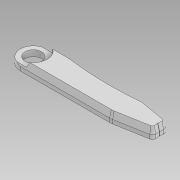
# Autodesk Inventor part: DoubleSlipHR_Bar
Saved by Autodesk Inventor 2021 (Build 250183000, 183)
## iProperties
Created: 2021-05-06
Part Number: DoubleSlipHR_Bar
Material: 一般
Document SubType Name: Modeling
Designer: kumagai
Density: 1 g/cm^3
Appearance: 既定
Author: kumagai
Autodesk Inventor part; units mm, degrees
ref_plane "YZ Plane" through (0, 0, 0) normal (1, 0, 0) x (0, 1, 0)
ref_plane "XZ Plane" through (0, 0, 0) normal (0, 1, 0) x (-1, 0, 0)
ref_plane "XY Plane" through (0, 0, 0) normal (0, 0, 1) x (1, 0, 0)
derived "DoubleSlipHR.ipt"
sketch "スケッチ1" plane through (0, 0, 0) normal (0, 1, 0) x (-1, 0, 0)
  line L0 (0, -123.3522) -> (0, 25.2475) projected
  line L1 (-47.4955, 0) -> (12.5826, 0) projected
  circle A0 centre (0, 0) radius 2.525
  circle A1 centre (0, 0) radius 4
  line L2 (0, 4) -> (-27.2419, 4)
  line L3 (-38.5128, 1.1628) -> (-38.4149, 0.0436)
  line L4 (-38.4149, -0.0436) -> (-38.5128, -1.1628)
  arc A2 (-38.4149, -0.0436) -> (-38.4149, 0.0436) centre (-38.913, 0) ccw
  arc A3 (-7.5002, -3.9826) -> (-29.3884, -3.5223) centre (-20.513, -102.1237) ccw
  line L5 (-31.474, 0) -> (-33.3295, 0)
  line L6 (0, -4) -> (-7.2374, -4)
  line L7 (-30.7049, -3.4665) -> (-37.6902, -2.2348)
  line L8 (-28.1101, 3.924) -> (-37.6902, 2.2348)
  arc A4 (-38.5128, -1.1628) -> (-37.6902, -2.2348) centre (-37.5166, -1.25) ccw
  arc A5 (-37.6902, 2.2348) -> (-38.5128, 1.1628) centre (-37.5166, 1.25) ccw
  arc A6 (-27.2419, 4) -> (-28.1101, 3.924) centre (-27.2419, -1) ccw
  arc A7 (-30.7049, -3.4665) -> (-29.3884, -3.5223) centre (-29.8366, 1.4575) ccw
  arc A8 (-7.5002, -3.9826) -> (-7.2374, -4) centre (-7.2374, -2) ccw
  point P0 (-38.411, 0)
  point P1 (-38.5278, -1.3348)
  point P2 (-38.4707, -0.6822)
  point P3 (-38.413, 0)
  point P4 (-31.0718, 4)
  point P5 (-7.37, -4)
  dimension "d1" = 5.05
  dimension "d2" = 8
  dimension "d4" = 0.5
  dimension "d7" = 170
  dimension "d9" = 38.413
  dimension "d14" = 20.513
  dimension "d15" = 102.1237
  dimension "d17" = 0
  dimension "d18" = 99
  dimension "d27" = 20
  dimension "d28" = 1
  dimension "d29" = 2.5
  dimension "d30" = 5
  dimension "d31" = 5
  dimension "d39" = 2
  constraints: 18 point on circle, 14 end point, 12 tangent, 10 point on line, 9 centre point, 3 horizontal, 2 coincident, 1 equal radius, 2 other
  measures "d1" diameter of A0
  measures "d2" diameter of A1
  measures "d4" radius of A2
  measures "d7" angle of L3 L4
  measures "d9" distance from line of point (-38.413, 0) L0
  measures "d14" distance from line of L0 A3.centre
  measures "d15" distance from line of L1 A3.centre
  measures "d17" distance between parallel lines of L1 L5
  measures "d18" radius of A3
  measures "d27" angle of L8 L7
  measures "d28" radius of A4
  measures "d29" distance of A5.centre A4.centre
  measures "d30" radius of A6
  measures "d31" radius of A7
  measures "d39" radius of A8
extrude "押し出し1" add sketch "スケッチ1" along normal blind 3.2 contours A1 L1 A0 L0 | L0 A0 L1 A1 | L6 A8 A3 A7 L7 A4 L4 A2 L1 A1 | L1 A0 L0 A1 | A1 L0 A0 L1 | L1 A2 L3 A5 L8 A6 L2 A1
sketch "スケッチ2" plane through (0, 3.2, 0) normal (0, 1, 0) x (1, 0, 0)
  circle A0 centre (0, 0) radius 2.525 projected
  circle A1 centre (0, 0) radius 4.25
  dimension "d24" = 8.5
  constraints: 1 centre point, 1 coincident
  measures "d24" diameter of A1
extrude "押し出し2" cut sketch "スケッチ2" against normal blind 1.4
chamfer "面取り1" distance 0.5 distance2 2 11 edges at (18.4315, 3.2, -3.1456) (30.0485, 3.2, -3.538) (34.1975, 3.2, -2.8507) (38.3099, 3.2, -1.8588) (38.4638, 3.2, -0.6032) (38.413, 3.2, 0) (38.4638, 3.2, 0.6032) (38.3099, 3.2, 1.8588) (32.9002, 3.2, 3.0794) (27.6777, 3.2, 3.981) (14.339, 3.2, 4) measured on face at (37.913, 3.2, 0) measured on face at (37.9133, 3.2, -1.5544) measured on face at (37.9657, 3.2, 0.6468) measured on face at (37.9657, 3.2, -0.6468) measured on face at (27.6341, 3.2, 3.4829) measured on face at (37.9133, 3.2, 1.5544) measured on face at (30.0273, 3.2, -3.0384) measured on face at (34.1107, 3.2, -2.3583) measured on face at (32.8134, 3.2, 2.587) measured on face at (14.339, 3.2, 3.5) measured on face at (18.421, 3.2, -2.6457)
equation "\"d9\" = exp_P1"
equation "\"d14\" = exp_P2"
equation "\"d15\" = exp_P3"
equation "\"d22\" = RailDepth"
equation "\"exp_P2\" = 20.513039"
equation "\"exp_P3\" = 102.123704"
equation "\"RailDepth\" = 3.2"
equation "\"exp_P1\" = 38.412951"
